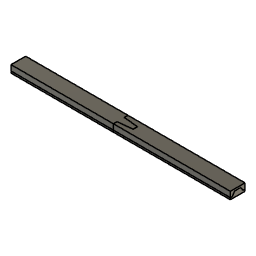
PoolHolder v3 (Autodesk Fusion 360 design; units mm, degrees)
Autodesk Fusion 360 part; units mm, degrees
note: some values were not read from the file. Chosen so that the rebuilt part matches the saved one: which bodies a step acts on; which face or edge a step refers to.
sketch "Skizze1" plane through (0, 0, 0) normal (0, 0, 1) x (1, 0, 0)
  line L0 (-75, 30) -> (225, 30)
  line L1 (225, 30) -> (225, 50)
  line L2 (225, 50) -> (-75, 50)
  line L3 (-75, 50) -> (-75, 30)
  line L4 (75, 55) -> (75, 25) construction
  dimension "d7" = 300
  dimension "d8" = 20
  constraint horizontal L0
  constraint vertical L1
  constraint horizontal L2
  constraint vertical L3
  constraint perpendicular L0 L4
  measures "d7" distance of L1.end L2.end
  measures "d8" distance of L0.start L2.end
extrude "Extrusion1" add sketch "Skizze1" along normal blind 10 makes body 1
sketch "Skizze6" plane through (0, 30, 0) normal (0, -1, 0) x (1, 0, 0)
  line L0 (-75, 0) -> (225, 0)
  line L1 (225, 0) -> (225, 10)
  line L2 (225, 10) -> (-75, 10)
  line L3 (-75, 10) -> (-75, 0)
  line L4 (-75, 10) -> (-75, 0) construction
  line L5 (-75, 5) -> (225, 5) construction
  dimension "d21" = 10
  dimension "d22" = 5
  constraint coincident L2.end L3.start
  constraint coincident L0.start L3.end
  constraint midpoint L4 L5.start
  constraint midpoint L1 L5.end
  measures "d21" distance of L2.end L0.start
  measures "d22" distance of L0 L5
sketch "Skizze8" plane through (-75, 0, 0) normal (-1, 0, 0) x (0, -1, 0)
  line L0 (-50, 0) -> (-30, 0)
  line L1 (-30, 0) -> (-30, 10)
  line L2 (-30, 10) -> (-50, 10)
  line L3 (-50, 10) -> (-50, 0)
  line L4 (-50, 5) -> (-30, 5) construction
  line L5 (-44, 7.5) -> (-36, 7.5)
  line L6 (-47.5, 2.5) -> (-44, 7.5)
  line L7 (-36, 7.5) -> (-32.5, 2.5)
  line L8 (-30, 2.5) -> (-32.5, 2.5)
  line L9 (-47.5, 2.5) -> (-50, 2.5)
  constraint midpoint L3 L4.start
  constraint midpoint L1 L4.end
  constraint perpendicular L3 L5
  constraint coincident L1 L8.start
  constraint perpendicular L1 L8
  constraint coincident L3 L9.end
  constraint perpendicular L3 L9
sketch "Skizze9" plane through (0, 0, 10) normal (0, 0, 1) x (-1, 0, 0)
  line L0 (75, -50) -> (75, -30)
  line L1 (75, -30) -> (-225, -30)
  line L2 (-225, -30) -> (-225, -50)
  line L3 (-225, -50) -> (75, -50)
  line L4 (-75, -50) -> (-75, -30) construction
  line L5 (-85, -43) -> (-85, -37)
  line L6 (-85, -43) -> (-65, -45)
  line L7 (-65, -45) -> (-65, -50)
  line L8 (-85, -37) -> (-65, -35)
  line L9 (-65, -35) -> (-65, -30)
  constraint midpoint L3 L4.start
  constraint midpoint L1 L4.end
  constraint perpendicular L3 L5
  constraint coincident L3 L7.end
  constraint perpendicular L3 L7
  constraint coincident L1 L9.end
  constraint perpendicular L1 L9
split "Teilen1" by curves path "Skizze9" along L7 L6 L5 L8 L9 bodies 1 makes body 2 at (178.3333, 39, 0)
split "Teilen2" by curves path "Skizze8" along L9 L6 L5 L7 L8 bodies 2 1 makes body 3 at (-28.3333, 38.3333, 10) makes body 4 at (178.3333, 39, 10)
extrude "Extrusion3" cut 4 faces at (65, 45.8333, 2.8571) (65, 48.3333, 6.1905) (65, 34.1667, 2.8571) (65, 31.6667, 6.1905) along direction (-1, 0, 0) blind 0.1 on bodies 1 3 bodies 1 3
extrude "Extrusion4" cut 2 faces at (75, 36, 2.5) (68.3333, 35.3333, 7.8571) along direction (-0.099504, 0.995037, 0) blind 0.1 on bodies 1 3 bodies 1 3
extrude "Extrusion5" cut 2 faces at (75, 44, 2.5) (68.3333, 44.6667, 7.8571) along direction (-0.099504, -0.995037, 0) blind 0.1 on bodies 1 3 bodies 1 3
extrude "Extrusion6" cut 2 faces at (85, 41, 2.5) (85, 41, 8.3333) along direction (-1, 0, 0) blind 0.1 on bodies 1 3 bodies 1 3
extrude "Extrusion7" cut 2 faces at (-25.335, 41.3333, 7.5) (178.3333, 41, 7.5) along direction (0, 0, -1) blind 0.1 on bodies 1 2 bodies 1 2
extrude "Extrusion8" cut 4 faces at (171.6667, 48.3333, 2.5) (-28.3667, 49.1667, 2.5) (171.6667, 30.8333, 2.5) (18.2667, 30.8333, 2.5) along direction (0, 0, -1) blind 0.1 on bodies 1 2 bodies 1 2
extrude "Extrusion9" cut 2 faces at (121.6667, 46.3333, 4.1667) (-28.3667, 45.5, 5.3571) along direction (0, -0.819232, -0.573462) blind 0.1 on bodies 1 2 bodies 1 2
extrude "Extrusion10" cut 2 faces at (121.6667, 33.6667, 4.1667) (-28.3667, 34.5, 5.3571) along direction (0, 0.819232, -0.573462) blind 0.1 on bodies 1 2 bodies 1 2
sketch "Skizze10" plane through (0, 0, 10) normal (0, 0, 1) x (-1, 0, 0)
  line L0 (-84.9, -37.0905) -> (-84.9, -42.9095)
  line L1 (-84.9, -42.9095) -> (-64.9901, -44.9005)
  line L2 (-64.9901, -44.9005) -> (-65, -45)
  line L3 (-65, -45) -> (-64.9, -45)
  line L4 (-64.9, -45) -> (-64.9, -50)
  line L5 (-64.9, -50) -> (75, -50)
  line L6 (75, -50) -> (75, -30)
  line L7 (75, -30) -> (-64.9, -30)
  line L8 (-64.9, -30) -> (-64.9, -35)
  line L9 (-64.9, -35) -> (-65, -35)
  line L10 (-65, -35) -> (-64.9901, -35.0995)
  line L11 (-64.9901, -35.0995) -> (-84.9, -37.0905)
  line L12 (75, -40) -> (-225, -40) construction
  circle A0 centre (35, -40) radius 2.55
  circle A1 centre (-24.9, -40) radius 2.55
  circle A2 centre (-104.9, -40) radius 2.55
  circle A3 centre (-185, -40) radius 2.55
  line L13 (-225, -30) -> (-225, -50) construction
  dimension "d39" = 5.1
  dimension "d40" = 5.1
  dimension "d41" = 5.1
  dimension "d42" = 5.1
  dimension "d43" = 139.9
  dimension "d44" = 140.1
  dimension "d45" = 40
  dimension "d46" = 40
  dimension "d48" = 40
  dimension "d49" = 59.9
  dimension "d51" = 80.1
  constraint midpoint L6 L12.start
  constraint perpendicular L8 L12
  constraint coincident L12 A0.centre
  constraint coincident L12 A1.centre
  constraint coincident L12 A2.centre
  constraint coincident L12 A3.centre
  measures "d39" diameter of A0
  measures "d40" diameter of A1
  measures "d41" diameter of A2
  measures "d42" diameter of A3
  measures "d43" distance of L4.end L5.end
  measures "d44" distance of L0 L13
  measures "d45" distance of L6 A0.centre
  measures "d46" distance of L4 A1.centre
  measures "d48" distance of A3.centre L13
  measures "d49" distance of A0.centre A1.centre
  measures "d51" distance of A2.centre A3.centre
extrude "Extrusion11" [rolled back] along distance -15 taper angle 0
sketch "Skizze11" plane through (0, 0, 10) normal (0, 0, 1) x (-1, 0, 0)
  circle A0 centre (-24.9, -40) radius 2.55
  circle A1 centre (35, -40) radius 2.55
  line L0 (-84.9, -37.0905) -> (-84.9, -42.9095)
  line L1 (-84.9, -42.9095) -> (-64.9901, -44.9005)
  line L2 (-64.9901, -44.9005) -> (-65, -45)
  line L3 (-65, -45) -> (-64.9, -45)
  line L4 (-64.9, -45) -> (-64.9, -50)
  line L5 (-64.9, -50) -> (75, -50)
  line L6 (75, -50) -> (75, -30)
  line L7 (75, -30) -> (-64.9, -30)
  line L8 (-64.9, -30) -> (-64.9, -35)
  line L9 (-64.9, -35) -> (-65, -35)
  line L10 (-65, -35) -> (-64.9901, -35.0995)
  line L11 (-64.9901, -35.0995) -> (-84.9, -37.0905)
  line L12 (35, -40) -> (-24.9, -40) construction
  line L13 (20.05, -45) -> (-9.95, -45)
  line L14 (-9.95, -45) -> (-9.95, -35)
  line L15 (-9.95, -35) -> (20.05, -35)
  line L16 (20.05, -35) -> (20.05, -45)
  line L17 (5.05, -35) -> (5.05, -30)
  line L18 (20.05, -40) -> (35, -40)
  dimension "d54" = 59.9
  dimension "d55" = 30
  dimension "d56" = 10
  dimension "d57" = 14.95
  dimension "d58" = 14.95
  constraint coincident A1.centre L12.start
  constraint coincident A0.centre L12.end
  constraint vertical L16
  constraint parallel L12 L15
  constraint parallel L12 L13
  constraint perpendicular L12 L14
  constraint midpoint L15 L17.start
  constraint midpoint L7 L17.end
  constraint vertical L17
  constraint midpoint L16 L18.start
  constraint horizontal L18
  measures "d54" distance of A1.centre A0.centre
  measures "d55" distance of L13.start L13.end
  measures "d56" distance of L13.start L15.end
  measures "d57" distance of A0.centre L14
  measures "d58" distance of A1.centre L16
